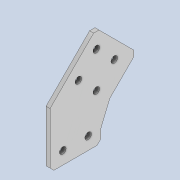
# Autodesk Inventor part: 45deg 2040 Connector Bracket
Saved by Autodesk Inventor 2022 (Build 260153000, 153)
## iProperties
Created: 2021-11-27
Part Number: 45deg 2040 Connector Bracket
Material: Generic
Document SubType Name: Modeling
Designer: Coy
Density: 1 g/cm^3
Appearance: Machined - Aluminum
Author: Coy
Autodesk Inventor part; units mm, degrees
ref_plane "YZ Plane" through (0, 0, 0) normal (1, 0, 0) x (0, 1, 0)
ref_plane "XZ Plane" through (0, 0, 0) normal (0, 1, 0) x (-1, 0, 0)
ref_plane "XY Plane" through (0, 0, 0) normal (0, 0, 1) x (1, 0, 0)
sketch "Sketch1" plane through (0, 0, 0) normal (1, 0, 0) x (0, 1, 0)
  line L0 (0, 0) -> (20, 0)
  line L1 (20, 0) -> (20, 40) construction
  line L2 (20, 40) -> (0, 40)
  line L3 (0, 40) -> (0, 0)
  line L4 (20, 0) -> (65, 0) construction
  line L5 (51.8198, 31.8198) -> (43.6396, 40)
  line L6 (43.6396, 40) -> (20, 40)
  line L7 (51.8198, 31.8198) -> (20, 0) construction
  line L8 (20, 0) -> (48.2843, -28.2843)
  line L9 (48.2843, -28.2843) -> (80.1041, 3.5355)
  line L10 (80.1041, 3.5355) -> (51.8198, 31.8198)
  line L11 (10, 40) -> (10, 0) construction
  circle A0 centre (10, 30) radius 2.6
  circle A1 centre (10, 10) radius 2.6
  line L12 (51.8198, 17.6777) -> (37.6777, 3.5355) construction
  line L13 (37.6777, 3.5355) -> (51.8198, -10.6066) construction
  line L14 (51.8198, -10.6066) -> (65.9619, 3.5355) construction
  line L15 (65.9619, 3.5355) -> (51.8198, 17.6777) construction
  circle A2 centre (65.9619, 3.5355) radius 2.6
  circle A3 centre (51.8198, 17.6777) radius 2.6
  circle A4 centre (37.6777, 3.5355) radius 2.6
  circle A5 centre (51.8198, -10.6066) radius 2.6
  dimension "d0" = 20
  dimension "d1" = 40
  dimension "d2" = 45
  dimension "d4" = 40
  dimension "d5" = 45
  dimension "d6" = 5.2
  dimension "d7" = 5.2
  dimension "d8" = 10
  dimension "d9" = 10
  dimension "d10" = 20
  dimension "d11" = 20
  dimension "d12" = 10
  dimension "d13" = 10
  dimension "d14" = 5.2
  dimension "d15" = 5.2
  dimension "d16" = 5.2
  dimension "d17" = 5.2
  constraints: 32 end point, 6 centre point, 6 parallel, 5 perpendicular, 4 coincident, 2 horizontal, 2 midpoint, 2 point on line
  measures "d0" distance of L2.end L1.end
  measures "d1" distance of L1.end L0.end
  measures "d2" distance of L0.end L5.start
  measures "d4" distance of L8.end L0.end
  measures "d5" angle of L4 L7
  measures "d6" diameter of A0
  measures "d7" diameter of A1
  measures "d8" distance from line of L2 A0.centre
  measures "d9" distance from line of L0 A1.centre
  measures "d10" distance of L13.end L12.end
  measures "d11" distance of L13.end L14.end
  measures "d12" distance between parallel lines of L10 L15
  measures "d13" distance between parallel lines of L7 L12
  measures "d14" diameter of A2
  measures "d15" diameter of A3
  measures "d16" diameter of A4
  measures "d17" diameter of A5
extrude "Extrusion1" add sketch "Sketch1" along normal blind 3.175
chamfer "Chamfer1" distance 10 angle 45 1 edges at (1.5875, 20, 0)
chamfer "Chamfer2" distance 3 angle 45 4 edges at (1.5875, 48.2843, -28.2843) (1.5875, 80.1041, 3.5355) (1.5875, 0, 0) (1.5875, 0, 40)
equation "\"d7\" = d6"
equation "\"d14\" = d6"
equation "\"d15\" = d6"
equation "\"d16\" = d6"
equation "\"d17\" = d6"
body "Solid1"
